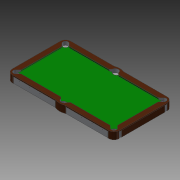
# Autodesk Inventor part: Table_Model
Saved by Autodesk Inventor 2015 (Build 190159000, 159)
## iProperties
Created: 2016-11-24
Part Number: Table_Model
Material: Generic
Document SubType Name: Modeling
Designer: Guy
Density: 1 g/cm^3
Appearance: Default
Author: Guy
Autodesk Inventor part; units mm, degrees
ref_plane "YZ Plane" through (0, 0, 0) normal (1, 0, 0) x (0, 1, 0)
ref_plane "XZ Plane" through (0, 0, 0) normal (0, 1, 0) x (-1, 0, 0)
ref_plane "XY Plane" through (0, 0, 0) normal (0, 0, 1) x (1, 0, 0)
sketch "Sketch1" plane through (0, 0, 0) normal (0, 0, 1) x (1, 0, 0)
  line L0 (0, 0) -> (2051, 0)
  line L1 (2051, 0) -> (2051, 1120.8)
  line L2 (2051, 1120.8) -> (0, 1120.8)
  line L3 (0, 1120.8) -> (0, 0)
  dimension "d0" = 2051
  dimension "d1" = 1120.8
  constraints: 8 end point, 2 parallel, 1 horizontal, 1 perpendicular
  measures "d0" distance of L2.end L1.end
  measures "d1" distance of L2.end L0.start
extrude "Extrusion1" add sketch "Sketch1" along normal blind 134.9
sketch "Sketch2" plane through (0, 0, 134.9) normal (0, 0, 1) x (1, 0, 0)
  line L0 (0, 0) -> (2051, 0) projected
  line L1 (2051, 0) -> (2051, 1120.8) projected
  line L2 (2051, 1120.8) -> (0, 1120.8) projected
  line L3 (0, 1120.8) -> (0, 0) projected
  line L4 (101.6, 100) -> (1949.4, 100)
  line L5 (1949.4, 100) -> (1949.4, 1020.8)
  line L6 (1949.4, 1020.8) -> (101.6, 1020.8)
  line L7 (101.6, 1020.8) -> (101.6, 100)
  dimension "d4" = 1847.8
  dimension "d5" = 920.8
  dimension "d6" = 101.6
  dimension "d7" = 100
  constraints: 8 end point, 2 parallel, 1 horizontal, 1 perpendicular
  measures "d4" distance of L5.end L6.end
  measures "d5" distance of L6.end L4.start
  measures "d6" distance between parallel lines of L3 L7
  measures "d7" distance between parallel lines of L0 L4
extrude "Extrusion2" cut sketch "Sketch2" against normal blind 39.7 contours L7 L6 L5 L4
ref_plane "Work Plane1" through (1025.5, 0, 0) normal (1, 0, 0) x (0, 0, -1)
sketch "Sketch4" plane through (1025.5, 0, 0) normal (1, 0, 0) x (0, 0, -1)
  line L0 (0, 1120.8) -> (0, 0) projected
  line L1 (0, 0) -> (-134.9, 0) projected
  line L2 (-134.9, 1120.8) -> (-134.9, 0) projected
  line L3 (0, 1120.8) -> (-134.9, 1120.8) projected
  line L4 (-134.9, 100) -> (-134.9, 1020.8) projected
  line L5 (-134.9, 100) -> (-134.9, 1020.8) projected
  line L6 (-134.9, 100) -> (-95.2, 100) projected
  line L7 (-95.2, 100) -> (-95.2, 1020.8) projected
  line L8 (-134.9, 1020.8) -> (-95.2, 1020.8) projected
  line L9 (-95.2, 100) -> (-95.2, 87.3)
  line L10 (-95.2, 87.3) -> (-126.96, 100)
  line L11 (-95.2, 1020.8) -> (-95.2, 1033.5)
  line L12 (-95.2, 1033.5) -> (-126.96, 1020.8)
  line L13 (-95.2, 1020.8) -> (-126.96, 1020.8)
  line L14 (-134.9, 1020.8) -> (-95.2, 1020.8) projected
  line L15 (-126.96, 100) -> (-95.2, 100)
  dimension "d20" = 12.7
  dimension "d21" = 7.94
  dimension "d22" = 12.7
  dimension "d23" = 7.94
  constraints: 12 end point, 3 point on line, 1 collinear, 1 horizontal, 1 vertical
  measures "d20" distance of L7.end L11.end
  measures "d21" distance from line of L12.end L2
  measures "d22" distance of L6.end L9.end
  measures "d23" distance of L4.start L10.end
extrude "Extrusion4" cut sketch "Sketch4" along normal mid plane 1848 contours L12 L11 L8 | L6 L9 L10
ref_plane "Work Plane2" through (0, 560.4, 0) normal (0, -1, 0) x (1, 0, 0)
sketch "Sketch6" plane through (0, 560.4, 0) normal (0, -1, 0) x (1, 0, 0)
  line L0 (2051, 0) -> (0, 0) projected
  line L1 (0, 0) -> (0, 134.9) projected
  line L2 (2051, 134.9) -> (0, 134.9) projected
  line L3 (2051, 0) -> (2051, 134.9) projected
  line L4 (101.6, 126.96) -> (101.6, 95.2) projected
  line L5 (101.6, 134.9) -> (101.6, 126.96) projected
  line L6 (1949.4, 134.9) -> (1949.4, 126.96) projected
  line L7 (1949.4, 126.96) -> (1949.4, 95.2) projected
  line L8 (1949.4, 95.2) -> (1962.1, 95.2)
  line L9 (1962.1, 95.2) -> (1949.4, 126.96)
  line L10 (1949.4, 126.96) -> (1949.4, 95.2)
  line L11 (101.6, 95.2) -> (88.9, 95.2)
  line L12 (88.9, 95.2) -> (101.6, 126.96)
  line L13 (101.6, 95.2) -> (101.6, 126.96)
  point P0 (0, 0)
  dimension "d39" = 12.7
  dimension "d40" = 12.7
  constraints: 12 end point, 2 collinear, 2 horizontal
  measures "d39" distance of L7.end L8.end
  measures "d40" distance of L4.end L11.end
extrude "Extrusion6" cut sketch "Sketch6" along normal mid plane 921 contours L4 L11 L12 | L9 L8 L7
sketch "Sketch7" plane through (0, 0, 134.9) normal (0, 0, 1) x (1, 0, 0)
  arc A0 (107.161, 1120.5433) -> (0.2098, 1014.3264) centre (100, 1020.8) ccw
  line L0 (0, 1120.8) -> (0, 0) projected
  line L1 (2051, 1120.8) -> (0, 1120.8) projected
  circle A1 centre (84.3045, 1036.5) radius 49.2
  line L2 (49.5197, 1071.2946) -> (29.2994, 1091.5207)
  line L3 (0, 1120.8) -> (0, 0) projected
  line L4 (0, 1020.8) -> (0, 1120.8)
  line L5 (0, 1120.8) -> (100, 1120.8)
  line L6 (1025.5, 1317.5448) -> (1025.5, -400.2984)
  line L7 (2051, 0) -> (2051, 1120.8) projected
  line L8 (2051, 1120.8) -> (2051, 0)
  line L9 (0, 1120.8) -> (2051, 1120.8)
  line L10 (-695.8087, 560.4) -> (2268.6576, 560.4)
  line L11 (0, 0) -> (2051, 0) projected
  line L12 (0, 0) -> (0, 1120.8)
  circle A2 centre (1966.7, 84.3045) radius 49.2
  arc A3 (1943.839, 0.2567) -> (2050.7902, 106.4736) centre (1951, 100) ccw
  line L13 (0, 0) -> (2051, 0)
  arc A4 (2051, 1020.8) -> (1951, 1120.8) centre (1951, 1020.8) ccw
  circle A5 centre (1966.7, 1036.4955) radius 49.2
  line L14 (2001.4946, 1071.2803) -> (2021.7207, 1091.5006)
  line L15 (2051, 1120.8) -> (1951, 1120.8)
  line L16 (2051, 1120.8) -> (0, 1120.8) projected
  line L17 (2051, 1120.8) -> (2051, 1020.8)
  line L18 (2051, 0) -> (2051, 1120.8) projected
  arc A6 (0, 100) -> (100, 0) centre (100, 100) ccw
  circle A7 centre (84.3, 84.3045) radius 49.2
  line L19 (49.5054, 49.5197) -> (29.2793, 29.2994)
  line L20 (0, 0) -> (100, 0)
  line L21 (0, 0) -> (0, 100)
  line L22 (2021.7207, 29.2994) -> (2001.4946, 49.5197)
  line L23 (2051, 0) -> (2051, 100)
  line L24 (2051, 0) -> (1951, 0)
  dimension "d45" = 98.4
  dimension "d63" = 98.4
  dimension "d64" = 98.4
  dimension "d68" = 98.4
  dimension "d43" = 100
  dimension "d44" = 28.6
  dimension "d46" = 84.3
  dimension "d47" = 84.3045
  dimension "d58" = 1025.5
  dimension "d59" = 560.4
  dimension "d60" = 100
  dimension "d61" = 28.6
  dimension "d62" = 84.3
  dimension "d65" = 28.6
  dimension "d66" = 84.3
  dimension "d67" = 100
  dimension "d69" = 28.6
  dimension "d70" = 100
  dimension "d71" = 84.3
  constraints: 36 end point, 18 point on circle, 9 point on line, 9 tangent, 6 symmetric about line, 4 centre point, 4 line through centre, 2 collinear, 2 parallel, 1 horizontal, 16 other
  measures "d43" radius of A0
  measures "d44" distance of L2.start L2.end
  measures "d46" distance from line of L1 point (84.304, 1036.5)
  measures "d47" distance from line of L0 point (84.304, 1036.5)
  measures "d58" distance between parallel lines of L6 L7
  measures "d59" distance between parallel lines of L11 L10
  measures "d60" radius of A4
  measures "d61" distance of L14.start L14.end
  measures "d62" distance from line of L7 point (1966.7, 1036.496)
  measures "d65" distance of L19.start L19.end
  measures "d66" distance from line of L0 point (84.3, 84.304)
  measures "d67" radius of A6
  measures "d69" distance of L22.start L22.end
  measures "d70" radius of A3
  measures "d71" distance from line of L8 point (1966.7, 84.304)
extrude "Extrusion7" cut sketch "Sketch7" against normal through all contours A0 L0 L1 | L1 L7 A4 | A6 L11 L0 | A3 L7 L11
extrude "Extrusion8" cut sketch "Sketch7" against normal blind 70 contours A1 | A2 | A5 | A7
sketch "Sketch8" plane through (0, 0, 134.9) normal (0, 0, 1) x (1, 0, 0)
  arc A0 (130.9322, 1020.8) -> (101.6, 990.4402) centre (84.3045, 1036.5) ccw projected
  line L0 (130.9322, 1020.8) -> (1920.0707, 1020.8) projected
  line L1 (1949.4, 990.4374) -> (1949.4, 130.3626) projected
  line L2 (1920.0707, 100) -> (130.9293, 100) projected
  line L3 (101.6, 130.3626) -> (101.6, 990.4402) projected
  arc A1 (100, 1120.8) -> (0, 1020.8) centre (100, 1020.8) ccw projected
  line L4 (0, 1020.8) -> (0, 100) projected
  line L5 (100, 0) -> (1951, 0) projected
  line L6 (2051, 100) -> (2051, 1020.8) projected
  line L7 (1951, 1120.8) -> (100, 1120.8) projected
  circle A2 centre (84.3045, 1036.5) radius 49.2 projected
  line L8 (118.7702, 1071.6106) -> (170.5314, 1020.8)
  arc A3 (130.9322, 1020.8) -> (101.6, 990.4402) centre (84.3045, 1036.5) ccw projected
  line L9 (130.9322, 1020.8) -> (170.5314, 1020.8)
  line L10 (130.9322, 1020.8) -> (1949.4, 1020.8) projected
  line L11 (101.6, 950.5788) -> (101.6, 990.4402)
  line L12 (101.6, 950.5788) -> (49.8387, 1001.3894)
  arc A4 (2051, 1020.8) -> (1951, 1120.8) centre (1951, 1020.8) ccw projected
  arc A5 (0, 100) -> (100, 0) centre (100, 100) ccw projected
  arc A6 (1951, 0) -> (2051, 100) centre (1951, 100) ccw projected
  arc A7 (1949.4, 990.4374) -> (1920.0707, 1020.8) centre (1966.7, 1036.4955) ccw projected
  arc A8 (1920.0707, 100) -> (1949.4, 130.3626) centre (1966.7, 84.3045) ccw projected
  arc A9 (101.6, 130.3626) -> (130.9293, 100) centre (84.3, 84.3045) ccw projected
  line L13 (1932.2361, 1071.6079) -> (1880.4722, 1020.8)
  line L14 (1920.0707, 1020.8) -> (1880.4722, 1020.8)
  arc A10 (1949.4, 990.4374) -> (1920.0707, 1020.8) centre (1966.7, 1036.4955) ccw projected
  line L15 (2001.1639, 1001.3832) -> (1949.4, 950.5753)
  line L16 (1949.4, 950.5753) -> (1949.4, 990.4374)
  line L17 (1949.4, 170.2247) -> (2001.1639, 119.4168)
  arc A11 (1920.0707, 100) -> (1949.4, 130.3626) centre (1966.7, 84.3045) ccw projected
  line L18 (1949.4, 170.2247) -> (1949.4, 130.3626)
  line L19 (1920.0707, 100) -> (1880.4722, 100)
  line L20 (1920.0707, 100) -> (130.9293, 100) projected
  line L21 (1880.4722, 100) -> (1932.2361, 49.1921)
  line L22 (101.6, 130.3626) -> (101.6, 170.2248)
  line L23 (101.6, 130.3626) -> (101.6, 990.4402) projected
  line L24 (101.6, 170.2248) -> (49.8361, 119.4168)
  line L25 (130.9293, 100) -> (170.5278, 100)
  line L26 (170.5278, 100) -> (118.7639, 49.1921)
  arc A12 (101.6, 130.3626) -> (130.9293, 100) centre (84.3, 84.3045) ccw projected
  point P0 (0, 0)
  dimension "d57" = 98.4
  dimension "d74" = 98.4
  dimension "d77" = 98.4
  dimension "d78" = 98.4
  constraints: 32 end point, 15 point on circle, 11 tangent, 10 point on line, 4 parallel, 2 collinear, 1 vertical
  measures "d57" distance of L8.end L11.start
  measures "d74" distance of L13.end L15.end
  measures "d77" distance of L17.start L19.end
  measures "d78" distance of L25.end L22.end
extrude "Extrusion9" cut sketch "Sketch8" against normal blind 39.7 contours A0 L8 L0 | L3 L12 A0 | L13 A7 L0 | L3 A9 L24 | L15 L1 A7 | A9 L2 L26 | L17 A8 L1 | L2 A8 L21
sketch "Sketch9" plane through (0, 0, 134.9) normal (0, 0, 1) x (1, 0, 0)
  arc A0 (2051, 1020.8) -> (1951, 1120.8) centre (1951, 1020.8) ccw projected
  line L0 (1951, 1120.8) -> (100, 1120.8) projected
  arc A1 (100, 1120.8) -> (0, 1020.8) centre (100, 1020.8) ccw projected
  line L1 (0, 1020.8) -> (0, 100) projected
  arc A2 (0, 100) -> (100, 0) centre (100, 100) ccw projected
  line L2 (100, 0) -> (1951, 0) projected
  arc A3 (1951, 0) -> (2051, 100) centre (1951, 100) ccw projected
  line L3 (2051, 100) -> (2051, 1020.8) projected
  line L4 (1949.4, 170.2247) -> (2001.1639, 119.4168) projected
  arc A4 (1932.2361, 49.1921) -> (2001.1639, 119.4168) centre (1966.7, 84.3045) ccw projected
  line L5 (1932.2361, 49.1921) -> (1880.4722, 100) projected
  line L6 (1880.4722, 100) -> (170.5278, 100) projected
  line L7 (170.5278, 100) -> (118.7639, 49.1921) projected
  arc A5 (49.8361, 119.4168) -> (118.7639, 49.1921) centre (84.3, 84.3045) ccw projected
  line L8 (49.8361, 119.4168) -> (101.6, 170.2248) projected
  line L9 (101.6, 170.2248) -> (101.6, 950.5788) projected
  line L10 (101.6, 950.5788) -> (49.8387, 1001.3894) projected
  arc A6 (118.7702, 1071.6106) -> (49.8387, 1001.3894) centre (84.3045, 1036.5) ccw projected
  line L11 (118.7702, 1071.6106) -> (170.5314, 1020.8) projected
  line L12 (170.5314, 1020.8) -> (1880.4722, 1020.8) projected
  line L13 (1880.4722, 1020.8) -> (1932.2361, 1071.6079) projected
  arc A7 (2001.1639, 1001.3832) -> (1932.2361, 1071.6079) centre (1966.7, 1036.4955) ccw projected
  line L14 (2001.1639, 1001.3832) -> (1949.4, 950.5753) projected
  line L15 (1949.4, 950.5753) -> (1949.4, 170.2247) projected
  line L16 (170.5314, 1020.8) -> (1880.4722, 1020.8) projected
  line L17 (934.2, 1020.8) -> (1116.8, 1020.8)
  line L18 (965, 1052.5) -> (1086, 1052.5)
  line L19 (965, 1052.5) -> (934.2, 1020.8)
  line L20 (1086, 1052.5) -> (1116.8, 1020.8)
  arc A8 (1116.8, 1120.8) -> (934.2, 1120.8) centre (1025.5, 901.605) ccw
  line L21 (1025.5, 1139.0542) -> (1025.5, 1110.4542)
  line L22 (1116.8, 1020.8) -> (1116.8, 1120.8)
  arc A9 (1086.1664, 1052.3287) -> (964.8336, 1052.3287) centre (1025.5, 1049.7322) ccw
  arc A10 (964.8336, 1052.3287) -> (1086.1664, 1052.3287) centre (1025.5, 1083.2434) ccw
  line L23 (1025.5, 1015.1542) -> (1025.5, 1110.4542)
  line L24 (-206.9931, 560.4) -> (2183.3755, 560.4)
  line L25 (965, 68.3) -> (1086, 68.3)
  line L26 (965, 68.3) -> (934.2, 100)
  line L27 (1086, 68.3) -> (1116.8, 100)
  arc A11 (934.2, 0) -> (1116.8, 0) centre (1025.5, 219.195) ccw
  line L28 (1025.5, -18.2542) -> (1025.5, 10.3458)
  line L29 (1116.8, 100) -> (1116.8, 0)
  arc A12 (964.8336, 68.4713) -> (1086.1664, 68.4713) centre (1025.5, 71.0678) ccw
  arc A13 (1086.1664, 68.4713) -> (964.8336, 68.4713) centre (1025.5, 37.5566) ccw
  line L30 (934.2, 100) -> (1116.8, 100)
  line L31 (1880.4722, 100) -> (170.5278, 100) projected
  line L32 (934.2, 0) -> (1116.8, 0)
  point P0 (0, 0)
  dimension "d81" = 182.6
  dimension "d82" = 121
  dimension "d84" = 31.7
  dimension "d86" = 28.6
  dimension "d92" = 95.3
  dimension "d95" = 560.4
  dimension "d96" = 28.6
  dimension "d97" = 31.7
  constraints: 30 end point, 17 point on circle, 13 symmetric about line, 8 point on line, 6 centre point, 2 collinear, 1 horizontal, 1 line through centre, 1 parallel, 1 perpendicular, 3 other
  measures "d81" distance of L17.start L17.end
  measures "d82" distance of L18.start L18.end
  measures "d84" distance between parallel lines of L17 L18
  measures "d86" distance of L21.start L21.end
  measures "d92" distance of L21.end L23.start
  measures "d95" distance between parallel lines of L2 L24
  measures "d96" distance of L28.start L28.end
  measures "d97" distance between parallel lines of L25 L6
extrude "Extrusion10" add sketch "Sketch9" against normal blind 134.9 contours L0 L21 A8 | L0 A8 L21 | A11 L28 L2 | L28 A11 L2
extrude "Extrusion11" cut sketch "Sketch9" against normal blind 39.7 contours L12 A10 L20 | L12 L23 L18 L20 A10 | A10 L12 L19 | L19 L18 L23 L12 A10 | L27 A13 L6 | A13 L27 L25 L26 L6 | L26 L6 A13
extrude "Extrusion12" cut sketch "Sketch9" against normal blind 70 contours L23 L18 L19 A9 | A9 L20 L18 L23 | A10 L23 L12 | L12 L23 L18 L20 A10 | L19 L18 L23 L12 A10 | L23 A10 L12 | A12 L26 L25 L27 | A13 L27 L25 L26 L6 | L6 A13
sketch "Sketch10" plane through (2051, 100, 0) normal (1, 0, 0) x (0, 0, -1)
  line L0 (0, 920.8) -> (-134.9, 920.8) projected
  line L1 (-134.9, 0) -> (-134.9, 920.8) projected
  line L2 (0, 0) -> (-134.9, 0) projected
  line L3 (0, 0) -> (0, 920.8) projected
  line L4 (-123.8, 43.7) -> (0, 43.7)
  line L5 (0, 43.7) -> (0, 877.1)
  line L6 (0, 877.1) -> (-123.8, 877.1)
  line L7 (-123.8, 877.1) -> (-123.8, 43.7)
  line L8 (0, 0) -> (0, 920.8) projected
  line L9 (-134.9, -118.2542) -> (0, -118.2542) projected
  line L10 (-134.9, 1039.0542) -> (0, 1039.0542) projected
  line L11 (0, -100) -> (-134.9, -100) projected
  line L12 (0, 1020.8) -> (-134.9, 1020.8) projected
  line L13 (-123.8, 43.7) -> (-123.8, 0)
  line L14 (-123.8, 877.1) -> (-123.8, 920.8)
  line L15 (-134.9, 920.8) -> (-123.8, 920.8)
  line L16 (0, 920.8) -> (-134.9, 920.8) projected
  line L17 (-134.9, 920.8) -> (-134.9, 0)
  line L18 (-134.9, 0) -> (-123.8, 0)
  line L19 (-123.8, 0) -> (0, 0)
  line L20 (0, 0) -> (0, 43.7)
  line L21 (0, 43.7) -> (-123.8, 43.7)
  line L22 (-123.8, 43.7) -> (-123.8, 0)
  line L23 (-123.8, 877.1) -> (0, 877.1)
  line L24 (0, 877.1) -> (0, 920.8)
  line L25 (0, 920.8) -> (-123.8, 920.8)
  line L26 (-123.8, 920.8) -> (-123.8, 877.1)
  dimension "d98" = 833.4
  dimension "d101" = 143.7
  dimension "d102" = 11.1
  constraints: 34 end point, 6 parallel, 4 collinear, 3 horizontal, 3 perpendicular, 2 point on line, 2 vertical
  measures "d98" distance of L6.end L4.start
  measures "d101" distance between parallel lines of L11 L4
  measures "d102" distance between parallel lines of L1 L7
extrude "Extrusion13" cut sketch "Sketch10" against normal blind 10 contours L3 L6 L14 L0 | L3 L2 L13 L4
extrude "Extrusion14" add sketch "Sketch10" along normal blind 10 contours L14 L7 L13 L2 L1 L0
ref_plane "Work Plane3" through (2051, 560.4, 134.9) normal (0, 1, 0) x (1, 0, 0)
sketch "Sketch11" plane through (2051, 560.4, 134.9) normal (0, 1, 0) x (1, 0, 0)
  line L0 (0, 11.1) -> (0, 0) projected
  line L1 (0, 11.1) -> (10, 11.1) projected
  line L2 (10, 0) -> (10, 11.1) projected
  line L3 (0, 0) -> (10, 0) projected
  arc A0 (0, 0) -> (10, 11.1) centre (-1.1605, 11.1) ccw
  line L4 (0, 0) -> (0, 11.1)
  line L5 (0, 11.1) -> (10, 11.1)
  line L6 (10, 11.1) -> (0, 11.1)
  point P0 (-2051, 134.9)
  constraints: 6 end point, 2 point on circle, 1 centre point, 1 collinear, 1 perpendicular, 1 tangent, 1 vertical
extrude "Extrusion15" cut sketch "Sketch11" along normal through all both and the other way through all contours A0 L2 L3
sketch "Sketch13" plane through (100, 0, 0) normal (0, -1, 0) x (1, 0, 0)
  line L0 (834.2, 0) -> (834.2, 134.9) projected
  line L1 (0, 134.9) -> (834.2, 134.9) projected
  line L2 (0, 0) -> (0, 134.9) projected
  line L3 (0, 0) -> (834.2, 0) projected
  line L4 (834.2, 134.9) -> (1016.8, 134.9) projected
  line L5 (834.2, 0) -> (834.2, 134.9) projected
  line L6 (1016.8, 0) -> (834.2, 0) projected
  line L7 (1016.8, 134.9) -> (1016.8, 0) projected
  line L8 (1016.8, 134.9) -> (1016.8, 0) projected
  line L9 (1016.8, 0) -> (1851, 0) projected
  line L10 (1851, 0) -> (1851, 134.9) projected
  line L11 (1016.8, 134.9) -> (1851, 134.9) projected
  line L12 (-100, 0) -> (-100, 134.9) projected
  line L13 (1951, 0) -> (1951, 123.8) projected
  line L14 (925.5, 445.4338) -> (925.5, -466.7984)
  circle A0 centre (125.5, 84.9) radius 4
  circle A1 centre (325.5, 84.9) radius 4
  circle A2 centre (525.5, 84.9) radius 4
  circle A3 centre (1325.5, 84.9) radius 4
  circle A4 centre (1525.5, 84.9) radius 4
  circle A5 centre (1725.5, 84.9) radius 4
  dimension "d114" = 1025.5
  dimension "d115" = 200
  dimension "d116" = 200
  dimension "d117" = 8
  dimension "d118" = 8
  dimension "d119" = 8
  dimension "d120" = 400
  dimension "d121" = 50
  dimension "d122" = 50
  dimension "d123" = 50
  dimension "d126" = 8
  dimension "d127" = 8
  dimension "d128" = 8
  dimension "d129" = 400
  dimension "d130" = 200
  dimension "d131" = 200
  dimension "d132" = 50
  dimension "d133" = 50
  dimension "d134" = 50
  constraints: 6 centre point, 2 end point, 1 vertical
  measures "d114" distance between parallel lines of L12 L14
  measures "d115" distance of A1.centre A2.centre
  measures "d116" distance of A0.centre A1.centre
  measures "d117" diameter of A2
  measures "d118" diameter of A1
  measures "d119" diameter of A0
  measures "d120" distance from line of A2.centre L14
  measures "d121" distance from line of L1 A2.centre
  measures "d122" distance from line of A1.centre L1
  measures "d123" distance from line of L1 A0.centre
  measures "d126" diameter of A3
  measures "d127" diameter of A4
  measures "d128" diameter of A5
  measures "d129" distance from line of L14 A3.centre
  measures "d130" distance of A3.centre A4.centre
  measures "d131" distance of A4.centre A5.centre
  measures "d132" distance from line of L11 A3.centre
  measures "d133" distance from line of L11 A4.centre
  measures "d134" distance from line of L11 A5.centre
extrude "Extrusion16" cut sketch "Sketch13" against normal blind 30 contours A0 | A1 | A2 | A3 | A4 | A5
sketch "Sketch14" plane through (100, 1120.8, 134.9) normal (0, 1, 0) x (1, 0, 0)
  line L0 (1016.8, 134.9) -> (1016.8, 0) projected
  line L1 (1851, 0) -> (1016.8, 0) projected
  line L2 (1851, 134.9) -> (1851, 0) projected
  line L3 (1851, 134.9) -> (1016.8, 134.9) projected
  line L4 (834.2, 0) -> (834.2, 134.9) projected
  line L5 (834.2, 134.9) -> (0, 134.9) projected
  line L6 (0, 134.9) -> (0, 0) projected
  line L7 (834.2, 0) -> (0, 0) projected
  line L8 (1951, 134.9) -> (1951, 11.1) projected
  line L9 (925.5, -179.8017) -> (925.5, 425.5685)
  circle A0 centre (1325.5, 50) radius 4
  circle A1 centre (1725.5, 50) radius 4
  circle A2 centre (1525.5, 50) radius 4
  circle A3 centre (525.5, 50) radius 4
  circle A4 centre (325.5, 50) radius 4
  circle A5 centre (125.5, 50) radius 4
  point P0 (-100, 134.9)
  dimension "d135" = 1025.5
  dimension "d136" = 400
  dimension "d137" = 200
  dimension "d138" = 200
  dimension "d139" = 8
  dimension "d140" = 8
  dimension "d141" = 8
  dimension "d142" = 50
  dimension "d143" = 50
  dimension "d144" = 50
  dimension "d145" = 400
  dimension "d146" = 200
  dimension "d148" = 200
  dimension "d149" = 8
  dimension "d150" = 8
  dimension "d151" = 8
  dimension "d152" = 50
  dimension "d153" = 50
  dimension "d154" = 50
  constraints: 6 centre point, 2 end point, 1 vertical
  measures "d135" distance between parallel lines of L8 L9
  measures "d136" distance from line of A0.centre L9
  measures "d137" distance of A2.centre A0.centre
  measures "d138" distance of A1.centre A2.centre
  measures "d139" diameter of A0
  measures "d140" diameter of A2
  measures "d141" diameter of A1
  measures "d142" distance from line of L1 A0.centre
  measures "d143" distance from line of L1 A2.centre
  measures "d144" distance from line of L1 A1.centre
  measures "d145" distance from line of L9 A3.centre
  measures "d146" distance of A3.centre A4.centre
  measures "d148" distance of A4.centre A5.centre
  measures "d149" diameter of A3
  measures "d150" diameter of A4
  measures "d151" diameter of A5
  measures "d152" distance from line of A3.centre L7
  measures "d153" distance from line of A4.centre L7
  measures "d154" distance from line of A5.centre L7
extrude "Extrusion17" cut sketch "Sketch14" against normal blind 30 contours A0 | A1 | A2 | A3 | A4 | A5
sketch "Sketch15" plane through (100, 1120.8, 134.9) normal (0, 1, 0) x (1, 0, 0)
  line L0 (834.2, 134.9) -> (0, 134.9) projected
  line L1 (820, 19.9) -> (20, 19.9)
  line L2 (20, 19.9) -> (20, 134.9)
  line L3 (20, 134.9) -> (820, 134.9)
  line L4 (820, 134.9) -> (820, 19.9)
  line L5 (0, 134.9) -> (0, 0) projected
  line L6 (1831, 134.9) -> (1031, 134.9)
  line L7 (1031, 134.9) -> (1031, 19.9)
  line L8 (1031, 19.9) -> (1831, 19.9)
  line L9 (1831, 19.9) -> (1831, 134.9)
  line L10 (1851, 134.9) -> (1016.8, 134.9) projected
  line L11 (1851, 134.9) -> (1851, 0) projected
  point P0 (-100, 134.9)
  dimension "d159" = 800
  dimension "d160" = 20
  dimension "d161" = 115
  dimension "d172" = 115
  dimension "d173" = 20
  dimension "d174" = 800
  constraints: 16 end point, 4 parallel, 2 horizontal, 2 perpendicular, 2 point on line
  measures "d159" distance of L1.start L1.end
  measures "d160" distance between parallel lines of L5 L2
  measures "d161" distance between parallel lines of L0 L1
  measures "d172" distance of L8.end L6.start
  measures "d173" distance between parallel lines of L11 L9
  measures "d174" distance of L7.end L8.end
extrude "Extrusion18" cut sketch "Sketch15" against normal blind 5.4
sketch "Sketch16" plane through (100, 0, 0) normal (0, -1, 0) x (1, 0, 0)
  line L0 (0, 0) -> (834.2, 0) projected
  line L1 (20, 0) -> (820, 0)
  line L2 (820, 0) -> (820, 115)
  line L3 (820, 115) -> (20, 115)
  line L4 (20, 115) -> (20, 0)
  line L5 (0, 0) -> (0, 134.9) projected
  line L6 (1031, 0) -> (1831, 0)
  line L7 (1831, 0) -> (1831, 115)
  line L8 (1831, 115) -> (1031, 115)
  line L9 (1031, 115) -> (1031, 0)
  line L10 (1016.8, 0) -> (1851, 0) projected
  line L11 (1851, 0) -> (1851, 134.9) projected
  point P0 (-100, 0)
  dimension "d164" = 20
  dimension "d165" = 800
  dimension "d166" = 115
  dimension "d167" = 20
  dimension "d168" = 800
  dimension "d169" = 115
  constraints: 16 end point, 4 parallel, 2 horizontal, 2 perpendicular, 2 point on line
  measures "d164" distance between parallel lines of L5 L4
  measures "d165" distance of L2.end L3.end
  measures "d166" distance between parallel lines of L0 L3
  measures "d167" distance between parallel lines of L11 L7
  measures "d168" distance of L7.end L8.end
  measures "d169" distance between parallel lines of L6 L8
extrude "Extrusion19" cut sketch "Sketch16" against normal blind 5.4
sketch "Sketch17" plane through (0, 0, 0) normal (0, 0, -1) x (-1, 0, 0)
  line L0 (-1931, 20.8) -> (-1131, 20.8)
  line L1 (-1131, 20.8) -> (-1131, 120.8)
  line L2 (-1131, 120.8) -> (-1931, 120.8)
  line L3 (-1931, 120.8) -> (-1931, 20.8)
  line L4 (-1931, 5.4) -> (-1131, 5.4) projected
  line L5 (-1131, 5.4) -> (-1131, 0) projected
  line L6 (-1931, 0) -> (-1931, 5.4) projected
  line L7 (-920, 20.8) -> (-120, 20.8)
  line L8 (-120, 20.8) -> (-120, 120.8)
  line L9 (-120, 120.8) -> (-920, 120.8)
  line L10 (-920, 120.8) -> (-920, 20.8)
  line L11 (-120, 5.4) -> (-120, 0) projected
  line L12 (-920, 0) -> (-920, 5.4) projected
  line L13 (-120, 0) -> (-920, 0) projected
  line L14 (-120, 0) -> (-120, 5.4) projected
  line L15 (-120, 5.4) -> (-920, 5.4) projected
  line L16 (-920, 0) -> (-920, 5.4) projected
  line L17 (-1931, 1000) -> (-1131, 1000)
  line L18 (-1131, 1000) -> (-1131, 1100)
  line L19 (-1131, 1100) -> (-1931, 1100)
  line L20 (-1931, 1100) -> (-1931, 1000)
  line L21 (-1131, 1120.8) -> (-1131, 1115.4) projected
  line L22 (-1931, 1115.4) -> (-1931, 1120.8) projected
  line L23 (-1131, 1115.4) -> (-1931, 1115.4) projected
  line L24 (-920, 1000) -> (-120, 1000)
  line L25 (-120, 1000) -> (-120, 1100)
  line L26 (-120, 1100) -> (-920, 1100)
  line L27 (-920, 1100) -> (-920, 1000)
  line L28 (-920, 1115.4) -> (-920, 1120.8) projected
  line L29 (-120, 1115.4) -> (-920, 1115.4) projected
  line L30 (-120, 1120.8) -> (-120, 1115.4) projected
  point P0 (0, 0)
  dimension "d175" = 15.4
  dimension "d176" = 100
  dimension "d177" = 15.4
  dimension "d178" = 100
  dimension "d179" = 15.4
  dimension "d180" = 100
  dimension "d181" = 15.4
  dimension "d182" = 100
  constraints: 32 end point, 8 collinear, 8 parallel, 4 horizontal, 4 perpendicular
  measures "d175" distance between parallel lines of L4 L0
  measures "d176" distance between parallel lines of L0 L2
  measures "d177" distance between parallel lines of L15 L7
  measures "d178" distance between parallel lines of L7 L9
  measures "d179" distance between parallel lines of L23 L19
  measures "d180" distance between parallel lines of L19 L17
  measures "d181" distance between parallel lines of L29 L26
  measures "d182" distance between parallel lines of L26 L24
extrude "Extrusion20" cut sketch "Sketch17" against normal blind 85 contours L3 L2 L1 L0 | L10 L9 L8 L7 | L20 L19 L18 L17 | L27 L26 L25 L24
body "Solid1"
